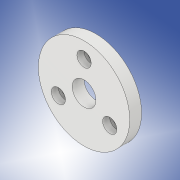
# Autodesk Inventor part: SJ018
Saved by Autodesk Inventor 2017 SP1 (Build 210196100, 196)
## iProperties
Created: 2017-07-25
Part Number: SJ018
Material: ABS Plastic
Document SubType Name: Modeling
Designer: Zach
Density: 1.06 g/cm^3
Appearance: CR White
Author: Zach
Autodesk Inventor part; units mm, degrees
ref_plane "YZ Plane" through (0, 0, 0) normal (1, 0, 0) x (0, 1, 0)
ref_plane "XZ Plane" through (0, 0, 0) normal (0, 1, 0) x (-1, 0, 0)
ref_plane "XY Plane" through (0, 0, 0) normal (0, 0, 1) x (1, 0, 0)
sketch "Sketch1" plane through (0, 0, 0) normal (0, 0, 1) x (1, 0, 0)
  circle A0 centre (0, 0) radius 19.25
  circle A1 centre (0, 12.5) radius 1.5
  circle A2 centre (-10.8253, -6.25) radius 1.5
  circle A3 centre (10.8253, -6.25) radius 1.5
  circle A4 centre (0, 0) radius 5
  dimension "d0" = 38.5
  dimension "d1" = 3
  dimension "d4" = 360
  dimension "d6" = 12.5
  dimension "d7" = 10
  constraints: 5 centre point, 2 coincident, 7 other
  measures "d0" diameter of A0
  measures "d1" diameter of A1
  measures "d6" distance of point (0, 0) A1.centre
  measures "d7" diameter of A4
extrude "Extrusion1" add sketch "Sketch1" along normal blind 5
sketch "Sketch2" plane through (0, 0, 5) normal (0, 0, 1) x (1, 0, 0)
  circle A0 centre (0, 12.5) radius 1.5 projected
  circle A1 centre (10.8253, -6.25) radius 1.5 projected
  circle A2 centre (-10.8253, -6.25) radius 1.5 projected
  circle A3 centre (0, 12.5) radius 3
  circle A4 centre (10.8253, -6.25) radius 1.5 projected
  circle A5 centre (10.8253, -6.25) radius 3
  circle A6 centre (-10.8253, -6.25) radius 3
  point P0 (0, 0)
  dimension "d10" = 6
  dimension "d11" = 6
  dimension "d12" = 6
  constraints: 3 centre point, 3 coincident
  measures "d10" diameter of A3
  measures "d11" diameter of A5
  measures "d12" diameter of A6
extrude "Extrusion2" cut sketch "Sketch2" against normal blind 3 contours A0 | A1 | A2 | A3 | A5 | A6
body "Solid1"
